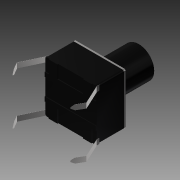
# Autodesk Inventor part: 6x6 mm
Saved by Autodesk Inventor 2014 SP2 (Build 180246200, 246)
## iProperties
Created: 2019-06-15
Part Number: 6x6 mm
Material: Generic
Document SubType Name: Modeling
Designer: Yuchofif
Density: 1 g/cm^3
Appearance: Steel - Polished
Author: Yuchofif
Autodesk Inventor part; units mm, degrees
ref_plane "YZ Plane" through (0, 0, 0) normal (1, 0, 0) x (0, 1, 0)
ref_plane "XZ Plane" through (0, 0, 0) normal (0, 1, 0) x (-1, 0, 0)
ref_plane "XY Plane" through (0, 0, 0) normal (0, 0, 1) x (1, 0, 0)
sketch "Sketch1" plane through (0, 0, 0) normal (0, 1, 0) x (-1, 0, 0)
  line L0 (3, 3) -> (-3, 3)
  line L1 (-3, 3) -> (-3, -3)
  line L2 (-3, -3) -> (3, -3)
  line L3 (3, -3) -> (3, 3)
  circle A0 centre (0, 0) radius 1.82
  constraints: 8 end point, 2 parallel, 1 centre point, 1 coincident, 1 horizontal, 1 perpendicular
extrude "Extrusion1" add sketch "Sketch1" against normal blind 3.4
sketch "Sketch2" plane through (0, 0, 0) normal (0, 1, 0) x (1, 0, 0)
  circle A0 centre (0, 0) radius 1.82 projected
  circle A1 centre (0, 0) radius 1.82
  constraints: 1 centre point, 1 coincident, 1 concentric
extrude "Extrusion2" add sketch "Sketch2" along normal blind 4.52 and the other way blind 3.4
sketch "Sketch3" plane through (0, 0, 0) normal (0, 1, 0) x (1, 0, 0)
  circle A0 centre (0, 0) radius 1.82 projected
  line L0 (-3, 3) -> (3, 3)
  line L1 (3, 3) -> (3, -3)
  line L2 (3, -3) -> (-3, -3)
  line L3 (-3, -3) -> (-3, 3)
  line L4 (-3, 3) -> (3, -3) construction
  line L5 (3, 3) -> (-3, -3) construction
  constraints: 12 end point, 2 midpoint, 2 parallel, 1 horizontal, 1 perpendicular
extrude "Extrusion3" add sketch "Sketch3" against normal blind 0.2
sketch "Sketch4" plane through (0, 0, 0) normal (0, 1, 0) x (1, 0, 0)
  circle A0 centre (0, 0) radius 1.82 projected
  line L0 (-3, -3) -> (3, -3) projected
  line L1 (3, -3) -> (3, 3) projected
  line L2 (3, 3) -> (-3, 3) projected
  line L3 (-3, 3) -> (-3, -3) projected
  line L4 (3.01, -3.01) -> (-3.01, -3.01)
  line L5 (-3.01, -3.01) -> (-3.01, 3.01)
  line L6 (-3.01, 3.01) -> (3.01, 3.01)
  line L7 (3.01, 3.01) -> (3.01, -3.01)
  line L8 (3.01, -3.01) -> (-3.01, 3.01) construction
  line L9 (-3.01, -3.01) -> (3.01, 3.01) construction
  constraints: 12 end point, 2 midpoint, 2 parallel, 1 horizontal, 1 perpendicular
extrude "Extrusion4" add sketch "Sketch4" against normal blind 0.2 contours L4 L5 L6 L7
sketch "Sketch5" plane through (0, 0, 0) normal (0, 1, 0) x (1, 0, 0)
  circle A0 centre (-2.26, 2.26) radius 0.62
  line L0 (3.01, -3.01) -> (-3.01, -3.01) projected
  line L1 (3.01, 3.01) -> (3.01, -3.01) projected
  line L2 (-3.01, 3.01) -> (3.01, 3.01) projected
  line L3 (-3.01, -3.01) -> (-3.01, 3.01) projected
  circle A1 centre (0, 0) radius 1.82 projected
  circle A2 centre (-2.26, -2.27) radius 0.62
  circle A3 centre (2.27, 2.26) radius 0.62
  circle A4 centre (2.27, -2.27) radius 0.62
  dimension "d22" = 4.53
  dimension "d25" = 4.53
  constraints: 4 centre point, 1 horizontal, 1 vertical, 6 other
  measures "d22" distance of A0.centre A2.centre
  measures "d25" distance of A0.centre A3.centre
extrude "Extrusion5" add sketch "Sketch5" along normal blind 0.2 contours A0 | A2 | A3 | A4
fillet "Fillet1" radius 0.2 4 edges at (3, -1.8, 3) (3, -1.8, -3) (-3, -1.8, -3) (-3, -1.8, 3)
fillet "Fillet2" radius 0.2 4 edges at (3.01, -0.1, 3.01) (-3.01, -0.1, 3.01) (-3.01, -0.1, -3.01) (3.01, -0.1, -3.01)
fillet "Fillet3" radius 0.2 4 edges at (1.65, 0.2, 2.27) (1.65, 0.2, -2.26) (-2.88, 0.2, -2.26) (-2.88, 0.2, 2.27)
sketch "Sketch6" plane through (-2.8, -3.4, 3) normal (0, 0, 1) x (1, 0, 0)
  line L0 (5.8, 0) -> (5.8, 3.2) projected
  line L1 (-0.2, 3.2) -> (-0.2, 0) projected
  line L2 (5.8, 0) -> (6.8565, -2.2658)
  line L3 (5.8, 0) -> (8.3, 0) construction
  line L4 (6.8565, -2.2658) -> (6.1065, -3.5648)
  line L5 (6.1065, -3.5648) -> (6.1265, -3.5648)
  line L6 (6.1265, -3.5648) -> (6.8765, -2.2658)
  line L7 (6.8765, -2.2658) -> (5.82, 0)
  line L8 (5.82, 0) -> (5.82, 0.3)
  line L9 (5.82, 0.3) -> (5.8, 0.3)
  line L10 (5.8, 0.3) -> (5.8, 0)
  line L11 (-0.2, 0) -> (-1.2565, -2.2658)
  line L12 (-1.2565, -2.2658) -> (-0.5065, -3.5648)
  line L13 (-0.5065, -3.5648) -> (-0.5265, -3.5648)
  line L14 (-0.5265, -3.5648) -> (-1.2765, -2.2658)
  line L15 (-1.2765, -2.2658) -> (-0.22, 0)
  line L16 (-0.22, 0) -> (-0.22, 0.3)
  line L17 (-0.22, 0.3) -> (-0.2, 0.3)
  line L18 (-0.2, 0.3) -> (-0.2, 0)
  point P0 (2.8, 3.4)
  constraints: 34 end point, 3 parallel, 2 point on line, 1 collinear, 1 equal length, 1 horizontal, 1 perpendicular
extrude "Extrusion6" add sketch "Sketch6" against normal blind 0.6
mirror "Mirror1" about plane through (0, 0, 0) normal (0, 0, 1) of "Extrusion6"
sketch "Sketch7" plane through (3.3265, -6.9648, 3) normal (0.8660254, -0.5, 0) x (0, 0, -1)
  line L0 (0.3, 0) -> (0.6, 0.5196)
  line L1 (0.3, 0) -> (0, 0.5196)
  line L2 (0.6, 0.5196) -> (0.6, 0)
  line L3 (0, 0) -> (0, 0.5196)
  line L4 (0.6, 0) -> (0.6, -0.0049)
  line L5 (0.6, -0.0049) -> (0, -0.0049)
  line L6 (0, -0.0049) -> (0, 0)
  point P0 (3, 4.3684)
  constraints: 14 end point, 2 parallel, 1 perpendicular
extrude "Extrusion7" cut sketch "Sketch7" against normal blind 0.6
sketch "Sketch8" plane through (3.3091, -6.9604, 3) normal (0.5, 0.8660254, 0) x (0.8660254, -0.5, 0)
  line L0 (0, 0) -> (0, 0.6) projected
  line L1 (0.0088, 0) -> (0, 0) projected
  line L2 (0.0088, 0.6) -> (0.0088, 0) projected
  line L3 (0, 0.6) -> (0.0088, 0.6) projected
  point P0 (-6.346, 3)
extrude "Extrusion8" cut sketch "Sketch8" against normal blind 0.6
fillet "Fillet4" radius 0.1 3 edges at (3.5789, -6.5105, 3) (3.319, -6.9605, 2.7) (3.5789, -6.5105, 2.4)
sketch "Sketch9" plane through (4.0765, -5.6658, -2.4) normal (0.8660254, -0.5, 0) x (0, 0, -1)
  line L0 (0.6, -1.5) -> (0.6, 0) projected
  line L1 (0, 0) -> (0, -1.5) projected
  line L2 (0.6, -1.5) -> (0, -1.5) projected
  line L3 (0.6, -1.51) -> (0, -1.51) projected
  line L4 (0.3, -1.5) -> (0.6, -0.9804)
  line L5 (0.3, -1.5) -> (0.5128, -1.5) construction
  line L6 (0.3, -1.5) -> (0, -0.9804)
  line L7 (0.6, -0.9804) -> (0.6, -1.5)
  line L8 (0.6, -1.5) -> (0, -1.5)
  line L9 (0, -1.5) -> (0, -0.9804)
  line L10 (0.6, -1.5) -> (0.6, -1.51)
  line L11 (0, -1.51) -> (0, -1.5)
  line L12 (0, -1.51) -> (0.6, -1.51)
  point P0 (-2.4, 2.8684)
  constraints: 18 end point, 3 parallel, 2 collinear, 2 point on line, 1 horizontal, 1 midpoint, 1 perpendicular
extrude "Extrusion9" cut sketch "Sketch9" against normal blind 0.6
fillet "Fillet5" radius 0.1 3 edges at (3.5789, -6.5105, -2.4) (3.319, -6.9605, -2.7) (3.5789, -6.5105, -3)
sketch "Sketch10" plane through (-4.0765, -5.6658, 2.4) normal (-0.8660254, -0.5, 0) x (0, 0, 1)
  line L0 (0.6, -1.5) -> (0.6, 0) projected
  line L1 (0, -1.5) -> (0, 0) projected
  line L2 (0.6, -1.51) -> (0, -1.51) projected
  line L3 (0.3, -1.5) -> (0.6, -0.9804)
  line L4 (0.3, -1.5) -> (0, -0.9804)
  line L5 (0.6, -1.5) -> (0, -1.5) projected
  line L6 (0.6, -0.9804) -> (0.6, -1.51)
  line L7 (0.6, -1.51) -> (0, -1.51)
  line L8 (0, -1.51) -> (0, -0.9804)
  line L9 (0, -1.5) -> (0.6, -1.5)
  point P0 (-2.4, 2.8684)
  constraints: 12 end point, 3 perpendicular, 2 point on line, 1 parallel
extrude "Extrusion10" cut sketch "Sketch10" against normal blind 0.6
fillet "Fillet6" radius 0.1 3 edges at (-3.5789, -6.5105, 3) (-3.319, -6.9605, 2.7) (-3.5789, -6.5105, 2.4)
sketch "Sketch11" plane through (-3.3265, -6.9648, -3) normal (-0.8660254, -0.5, 0) x (0, 0, 1)
  line L0 (0, 0) -> (0, 1.5) projected
  line L1 (0.6, 0) -> (0.6, 1.5) projected
  line L2 (0, -0.01) -> (0.6, -0.01) projected
  line L3 (0.3, 0) -> (0.6, 0.5196)
  line L4 (0.3, 0) -> (0, 0.5196)
  line L5 (0, 0) -> (0.6, 0) projected
  line L6 (0.6, 0.5196) -> (0.6, -0.01)
  line L7 (0.6, -0.01) -> (0, -0.01)
  line L8 (0, -0.01) -> (0, 0.5196)
  line L9 (0, 0) -> (0.6, 0)
  point P0 (3, 4.3684)
  constraints: 12 end point, 2 collinear, 2 point on line, 1 parallel, 1 perpendicular
extrude "Extrusion11" cut sketch "Sketch11" against normal blind 0.6
fillet "Fillet7" radius 0.1 3 edges at (-3.319, -6.9605, -2.7) (-3.5789, -6.5105, -2.4) (-3.5789, -6.5105, -3)
sketch "Sketch12" plane through (0, -3.4, 0) normal (0, -1, 0) x (1, 0, 0)
  line L0 (-3, 1) -> (3, 1)
  line L1 (3, 1) -> (3, 1.5)
  line L2 (-3, 1.5) -> (-3, 1)
  line L3 (-1.5, 1.5) -> (-1.5, 3)
  line L4 (-1.5, 3) -> (-2.5, 3)
  line L5 (-2.5, 3) -> (-2.5, 1.5)
  line L6 (3, 1.5) -> (2.5, 1.5)
  line L7 (1.5, 1.5) -> (1.5, 3)
  line L8 (1.5, 3) -> (2.5, 3)
  line L9 (2.5, 3) -> (2.5, 1.5)
  line L10 (3, 1.5) -> (2.5, 1.5)
  line L11 (1.5, 1.5) -> (-1.5, 1.5)
  line L12 (-2.5, 1.5) -> (-3, 1.5)
  line L13 (0, 0) -> (0.5123, 0)
  line L14 (-3, -1) -> (3, -1)
  line L15 (3, -1) -> (3, -1.5)
  line L16 (-3, -1.5) -> (-3, -1)
  line L17 (-1.5, -1.5) -> (-1.5, -3)
  line L18 (-1.5, -3) -> (-2.5, -3)
  line L19 (-2.5, -3) -> (-2.5, -1.5)
  line L20 (1.5, -1.5) -> (1.5, -3)
  line L21 (1.5, -3) -> (2.5, -3)
  line L22 (2.5, -3) -> (2.5, -1.5)
  line L23 (3, -1.5) -> (2.5, -1.5)
  line L24 (1.5, -1.5) -> (-1.5, -1.5)
  line L25 (-2.5, -1.5) -> (-3, -1.5)
  constraints: 52 end point, 12 symmetric about line, 7 parallel, 1 horizontal, 1 perpendicular
extrude "Extrusion12" add sketch "Sketch12" along normal blind 0.1
body "Solid1"
